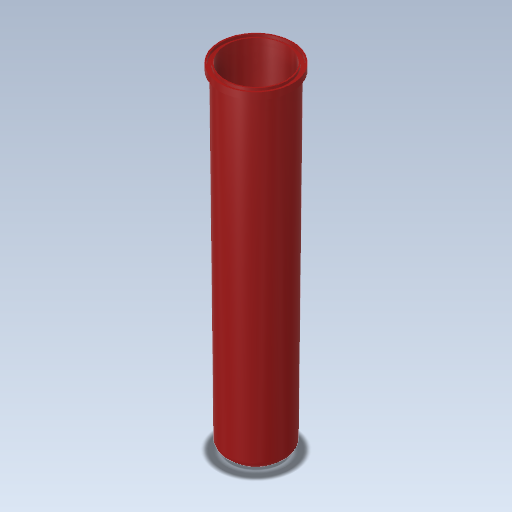
# Autodesk Inventor part: Filtr HOT 3P -dzwon
Saved by Autodesk Inventor 2020 (Build 240168000, 168)
## iProperties
Created: 2019-03-28
Part Number: Filtr HOT 3P -dzwon
Material: Tworzywo sztuczne PBT
Document SubType Name: Modeling
Designer: Marcin Kret
Mass: 850.3 g
Surface Area: 2916.51 cm^2
Volume: 649.084 cm^3
Density: 1.31 g/cm^3
Appearance: Czerwona
Author: Marcin Kret
Autodesk Inventor part; units mm, degrees
ref_plane "YZ Plane" through (0, 0, 0) normal (1, 0, 0) x (0, 1, 0)
ref_plane "XZ Plane" through (0, 0, 0) normal (0, 1, 0) x (-1, 0, 0)
ref_plane "XY Plane" through (0, 0, 0) normal (0, 0, 1) x (1, 0, 0)
sketch "Szkic1" plane through (0, 0, 0) normal (0, 0, 1) x (1, 0, 0)
  line L0 (0, 0) -> (-49, 0)
  line L1 (-49, 0) -> (-44.734207, -469.237256)
  arc A0 (-44.734207, -469.237256) -> (-34.824152, -480.944861) centre (-32.734703, -469.12817) ccw
  arc A1 (-34.824152, -480.944861) -> (0, -484) centre (0, -284) ccw
  line L2 (-49, 0) -> (-54, 0)
  line L3 (-54, 0) -> (-54, 10)
  line L4 (-54, 10) -> (0, 10)
  line L5 (0, 10) -> (0, 0)
  line L6 (0, 0) -> (0, -484)
  line L7 (-45, -440) -> (0, -440) construction
  line L8 (-33.5, -481.174415) -> (-32.721033, -484.081559)
  arc A2 (-32.721033, -484.081559) -> (-30.264387, -483.80166) centre (-31.513626, -483.758035) ccw
  line L9 (-30.264387, -483.80166) -> (-30.191278, -481.708085)
  line L10 (0, -485) -> (-31.372122, -485) construction
  line L11 (-51.5, 10) -> (-46.5, 10)
  line L12 (-46.5, 10) -> (-46.5, 6)
  line L13 (-46.5, 6) -> (-51.5, 6)
  line L14 (-51.5, 6) -> (-51.5, 10)
  dimension "d0" = 494
  dimension "d1" = 108
  dimension "d2" = 10
  dimension "d3" = 98
  dimension "d4" = 44
  dimension "d5" = 90
  dimension "d6" = 12
  dimension "d7" = 200
  dimension "d8" = 1
  dimension "d9" = 67
  dimension "d10" = 1.25
  dimension "d11" = 2
  dimension "d12" = 15
  dimension "d15" = 103
  dimension "d16" = 93
  dimension "d17" = 4
  constraints: 30 end point, 9 point on circle, 5 perpendicular, 4 horizontal, 4 tangent, 3 centre point, 3 point on line, 3 vertical alignment, 2 parallel, 1 vertical
  measures "d0" distance from line of L6.end L4
  measures "d1" diameter of L3 L6
  measures "d2" distance of L2.end L3.end
  measures "d3" diameter of L0.end L6
  measures "d4" distance from line of L6.end L7
  measures "d5" diameter of L7.start L6
  measures "d6" radius of A0
  measures "d7" radius of A1
  measures "d8" distance from line of L6.end L10
  measures "d9" diameter of L8.start L6
  measures "d10" radius of A2
  measures "d11" angle of L6 L9
  measures "d12" angle of L6 L8
  measures "d15" diameter of L14 L6
  measures "d16" diameter of L12 L6
  measures "d17" distance between parallel lines of L13 L4
revolve "Obrót1" add sketch "Szkic1" angle 360 about axis through (0, 0, 0) along (0, -1, 0) contours L6 A1 A0 L1 L0
shell "Skorupa1" thickness 4.5 removed faces 1 at (-6.635491, 0, 7.692832)
revolve "Obrót2" add sketch "Szkic1" angle 360 about axis through (0, 0, 0) along (0, -1, 0) contours L0 L2 L3 L4 L14 L13 L12 L5
sketch "Szkic2" plane through (0, 0, 0) normal (0, -1, 0) x (1, 0, 0)
  circle A0 centre (0, 0) radius 44.499814
extrude "Wyciągnięcie proste1" cut sketch "Szkic2" against normal through all
revolve "Obrót3" add sketch "Szkic1" angle 360 about axis through (0, 0, 0) along (0, -1, 0) contours L9 A2 L8 A1
